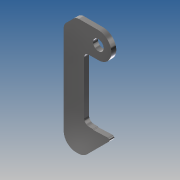
# Autodesk Inventor part: DD_KVD_002_07
Saved by Autodesk Inventor 2017.3 (Build 213256000, 256)
## iProperties
Created: 2023-11-02
Part Number: DD_KVD_002_07
Material: Nerezová ocel
Document SubType Name: Sheet Metal
Designer: Darena
Density: 8 g/cm^3
Sheet Metal Rule: Výchozí_mm
Appearance: Pololeštěná
Flat Pattern Width: 14.35 cm
Flat Pattern Length: 5.85 cm
Flat Pattern Area: 83.9475 cm^2
Sheet Metal Width: 143,500 mm
Sheet Metal Length: 58,500 mm
Sheet Metal Area: 8394,750 mm^2
Author: Darena
Autodesk Inventor part; units mm, degrees
ref_plane "YZ Plane" through (0, 0, 0) normal (1, 0, 0) x (0, 1, 0)
ref_plane "XZ Plane" through (0, 0, 0) normal (0, 1, 0) x (-1, 0, 0)
ref_plane "XY Plane" through (0, 0, 0) normal (0, 0, 1) x (1, 0, 0)
sketch "Náčrt2" plane through (0, 0, 0) normal (0, 1, 0) x (-1, 0, 0)
  line L0 (11.5, 17.5) -> (-11.5, 17.5) construction
  line L1 (-17.5, 11.5) -> (-17.5, -11.5) construction
  line L2 (-11.5, -17.5) -> (11.5, -17.5) construction
  line L3 (17.5, -11.5) -> (17.5, 11.5) construction
  line L4 (42.5, 36) -> (42.5, -77.5)
  line L5 (9, -22.5) -> (-14, -22.5) construction
  line L6 (-20, -28.5) -> (-20, -51.5) construction
  line L7 (-14, -57.5) -> (9, -57.5) construction
  line L8 (15, -51.5) -> (15, -28.5) construction
  arc A0 (15, -28.5) -> (9, -22.5) centre (9, -28.5) ccw construction
  arc A1 (9, -57.5) -> (15, -51.5) centre (9, -51.5) ccw construction
  arc A2 (-20, -51.5) -> (-14, -57.5) centre (-14, -51.5) ccw construction
  arc A3 (-14, -22.5) -> (-20, -28.5) centre (-14, -28.5) ccw construction
  line L9 (-45.6938, -20) -> (9, -20) construction
  arc A4 (17.5, -28.5) -> (9, -20) centre (9, -28.5) ccw construction
  line L10 (17.5, -28.5) -> (17.5, -51.5) construction
  line L11 (17.5, -51.5) -> (15, -51.5) construction
  line L12 (-14, -22.5) -> (-45.6938, -22.5) construction
  line L13 (-45.6938, -22.5) -> (-45.6938, -20) construction
  arc A5 (17.5, 11.5) -> (11.5, 17.5) centre (11.5, 11.5) ccw construction
  arc A6 (11.5, -17.5) -> (17.5, -11.5) centre (11.5, -11.5) ccw construction
  arc A7 (-17.5, -11.5) -> (-11.5, -17.5) centre (-11.5, -11.5) ccw construction
  arc A8 (-11.5, 17.5) -> (-17.5, 11.5) centre (-11.5, 11.5) ccw construction
  line L14 (-11.5, -20) -> (11.5, -20) construction
  line L15 (-20, 73.4113) -> (-20, -11.5) construction
  arc A9 (-20, -11.5) -> (-11.5, -20) centre (-11.5, -11.5) ccw construction
  line L16 (-17.5, 11.5) -> (-17.5, 73.4113) construction
  line L17 (-17.5, 73.4113) -> (-20, 73.4113) construction
  line L18 (11.5, -20) -> (11.5, -17.5) construction
  line L19 (17.5, 17.5) -> (-17.5, 17.5) construction
  line L20 (-17.5, 17.5) -> (-17.5, 52.5) construction
  line L21 (-17.5, 52.5) -> (17.5, 52.5) construction
  line L22 (17.5, 52.5) -> (17.5, 17.5) construction
  circle A10 centre (0, 35) radius 6.5
  arc A11 (0, 51) -> (0, 19) centre (0, 35) ccw
  line L23 (0, 51) -> (27.5, 51)
  line L24 (0, 19) -> (11.5, 19)
  line L25 (27.5, 51) -> (42.5, 36)
  arc A12 (17.5, 13) -> (11.5, 19) centre (11.5, 13) ccw
  line L26 (17.5, 13) -> (17.5, -51.5)
  line L27 (-13.5, -57.5) -> (-13.5, -59.2574)
  line L28 (-12.6213, -61.3787) -> (14.1066, -88.1066)
  line L29 (24.7132, -92.5) -> (27.5, -92.5)
  arc A13 (27.5, -92.5) -> (42.5, -77.5) centre (27.5, -77.5) ccw
  arc A14 (14.1066, -88.1066) -> (24.7132, -92.5) centre (24.7132, -77.5) ccw
  arc A15 (-13.5, -59.2574) -> (-12.6213, -61.3787) centre (-10.5, -59.2574) ccw
  line L30 (17.5, -51.5) -> (17.5, -51.5)
  line L31 (6.4677, -58.2408) -> (-10.5, -57.5)
  line L32 (-13.5, -57.5) -> (-10.5, -57.5)
  line L33 (6.4677, -58.2408) -> (6.5, -57.5)
  line L34 (6.5, -57.5) -> (11.5, -57.5)
  arc A16 (11.5, -57.5) -> (17.5, -51.5) centre (11.5, -51.5) ccw
  point P0 (0, 0)
  point P1 (17.5, 0)
  point P2 (0, 17.5)
  point P3 (42.5, 51)
  point P4 (17.5, 35)
  point P5 (0, 52.5)
  point P6 (-13.5, -60.5)
  dimension "d34" = 35
  dimension "d35" = 6
  dimension "d36" = 5
  dimension "d37" = 2.5
  dimension "d38" = 2.5
  dimension "d39" = 6
  dimension "d40" = 2.5
  dimension "d43" = 25
  dimension "d46" = 13
  dimension "d47" = 32
  dimension "d48" = 15
  dimension "d49" = 15
  dimension "d50" = 6
  dimension "d51" = 35
  dimension "d55" = 3
  dimension "d56" = 15
  dimension "d57" = 15
  dimension "d58" = 3
  dimension "d60" = 35
  dimension "d61" = 3
  dimension "d62" = 2.5
  dimension "d63" = 35
  dimension "d64" = 45
  dimension "d66" = 31
  dimension "d69" = 6
  dimension "d72" = 2.5
  constraints: 70 end point, 33 point on circle, 28 tangent, 17 centre point, 10 perpendicular, 10 point on line, 7 parallel, 6 equal radius, 5 collinear, 5 horizontal, 4 midpoint, 4 vertical, 2 horizontal alignment, 2 vertical alignment, 1 coincident, 3 other
  measures "d34" distance between parallel lines of L7 L5
  measures "d35" radius of A0
  measures "d36" distance between parallel lines of L2 L5
  measures "d37" distance between parallel lines of L1 L6
  measures "d38" distance between parallel lines of L5 L9
  measures "d39" radius of A5
  measures "d40" radial gap between concentric circles of A7 A9
  measures "d43" distance between parallel lines of L4 L10
  measures "d46" diameter of A10
  measures "d47" diameter of A11
  measures "d48" distance of L23.end point (42.5, 51)
  measures "d49" distance of L4.start point (42.5, 51)
  measures "d50" radius of A12
  measures "d51" distance between parallel lines of L0 L2
  measures "d55" distance of L27.start point (-13.5, -60.5)
  measures "d56" radius of A13
  measures "d57" radius of A14
  measures "d58" radius of A15
  measures "d60" distance between parallel lines of L1 L3
  measures "d61" distance of L27.start L31.end
  measures "d62" angle of L31 L7
  measures "d63" distance between parallel lines of L29 L7
  measures "d64" angle of L28 L7
  measures "d66" distance from line of L27.start L26
  measures "d69" radius of A16
  measures "d72" distance of L33.end L7.end
extrude "Vysunutí1" add sketch "Náčrt2" along normal blind 6
fillet "Zaoblení3" radius 2 1 edges at (13.5, 3, -57.5)
fillet "Zaoblení4" radius 10 2 edges at (-27.5, 3, 51) (-42.5, 3, 36)
fillet "Zaoblení5" radius 1 2 edges at (-6.5, 3, -57.5) (-6.4677, 3, -58.2408)
equation "\"d49\" = d48"
equation "\"PoloměrOhybu\" = Tloušťka"
equation "\"ŠířkaVýštipu\" = Tloušťka"
equation "\"HloubkaVýštipu\" = 0.5 * Tloušťka"
equation "\"VelikostRohovéhoVýštipu\" = 4 * Tloušťka"
equation "\"MinimálníZbytek\" = 2 * Tloušťka"
equation "\"PřechodovýPoloměr\" = PoloměrOhybu"
equation "\"VelikostJacobihoPoloměru\" = PoloměrOhybu"
equation "\"VelikostMezery\" = Tloušťka"
equation "\"Tloušťka\" = 6"
